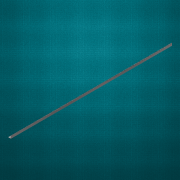
# Autodesk Inventor part: Metal Rail
Saved by Autodesk Inventor 2017 (Build 210142000, 142)
## iProperties
Created: 2017-09-04
Part Number: Metal Rail
Material: Steel, Galvanized
Document SubType Name: Modeling
Designer: Michael
Density: 7.85 g/cm^3
Appearance: Galvanized
Author: Michael
Autodesk Inventor part; units mm, degrees
ref_plane "YZ Plane" through (0, 0, 0) normal (1, 0, 0) x (0, 1, 0)
ref_plane "XZ Plane" through (0, 0, 0) normal (0, 1, 0) x (-1, 0, 0)
ref_plane "XY Plane" through (0, 0, 0) normal (0, 0, 1) x (1, 0, 0)
sketch "Sketch1" plane through (0, 0, 0) normal (0, 0, 1) x (1, 0, 0)
  arc A0 (-31.75, 3.175) -> (-34.925, 0) centre (-31.75, 0) ccw
  line L0 (-31.75, 3.175) -> (-1.5875, 3.175)
  line L1 (-1.5875, 3.175) -> (-1.5875, 27.5499)
  arc A1 (-1.5875, 27.5499) -> (-2.3813, 29.6499) centre (-4.7625, 27.5499) ccw
  line L2 (-34.925, 0) -> (-33.3375, 0)
  arc A2 (-31.75, 1.5875) -> (-33.3375, 0) centre (-31.75, 0) ccw
  line L3 (-31.75, 1.5875) -> (0, 1.5875)
  line L4 (0, 1.5875) -> (0, 27.5499)
  arc A3 (0, 34.925) -> (-2.3813, 29.6499) centre (0, 31.75) ccw
  arc A4 (0, 27.5499) -> (-1.1906, 30.7) centre (-4.7625, 27.5499) ccw
  arc A5 (0, 33.3375) -> (-1.1906, 30.7) centre (0, 31.75) ccw
  line L5 (0, 34.925) -> (0, 33.3375)
  point P0 (0, 0)
  dimension "d0" = 34.925
  dimension "d1" = 1.5875
  dimension "d2" = 1.5875
  dimension "d4" = 3.175
  dimension "d5" = 3.175
  dimension "d6" = 34.925
  dimension "d7" = 3.175
  dimension "d8" = 1.5875
  constraints: 12 end point, 12 point on circle, 6 centre point, 6 tangent, 3 coincident, 3 horizontal, 3 point on line, 2 perpendicular, 1 horizontal alignment, 1 vertical
  measures "d0" distance of L2.start point (0, 0)
  measures "d1" distance between parallel lines of L3 L0
  measures "d2" distance between parallel lines of L4 L1
  measures "d4" radius of A3
  measures "d5" radius of A0
  measures "d6" distance of point (0, 0) L5.start
  measures "d7" radius of A1
  measures "d8" distance centre to line of A3 L1
extrude "Extrusion1" add sketch "Sketch1" along normal mid plane 2003.425
body "Solid1"
